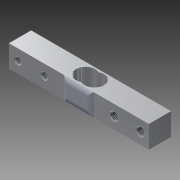
# Autodesk Inventor part: Weight Sensor
Saved by Autodesk Inventor 2014 SP1 (Build 180222100, 222)
## iProperties
Created: 2015-08-12
Part Number: Weight Sensor
Material: Алюминий 6061-AHC
Document SubType Name: Modeling
Designer: romanov.mv
Density: 2.71 g/cm^3
Appearance: Алюминий — темный
Author: romanov.mv
Autodesk Inventor part; units mm, degrees
ref_plane "YZ Plane" through (0, 0, 0) normal (1, 0, 0) x (0, 1, 0)
ref_plane "XZ Plane" through (0, 0, 0) normal (0, 1, 0) x (-1, 0, 0)
ref_plane "XY Plane" through (0, 0, 0) normal (0, 0, 1) x (1, 0, 0)
sketch "Эскиз1" plane through (0, 0, 0) normal (0, 1, 0) x (-1, 0, 0)
  line L0 (-40, 6.35) -> (40, 6.35)
  line L1 (40, 6.35) -> (40, -6.35)
  line L2 (40, -6.35) -> (-40, -6.35)
  line L3 (-40, -6.35) -> (-40, 6.35)
  line L4 (-40, 6.35) -> (40, -6.35) construction
  line L5 (40, 6.35) -> (-40, -6.35) construction
  point P0 (0, 0)
  dimension "d0" = 80
  dimension "d1" = 12.7
  constraints: 12 end point, 2 midpoint, 2 parallel, 1 horizontal, 1 perpendicular
  measures "d0" distance of L1.end L2.end
  measures "d1" distance of L0.end L1.end
extrude "Выдавливание1" add sketch "Эскиз1" along normal blind 12.7
sketch "Эскиз2" plane through (0, 12.7, 0) normal (0, 1, 0) x (1, 0, 0)
  point P0 (0, 0)
  point P1 (-35, 0)
  point P2 (-20, 0)
  point P3 (20, 0)
  point P4 (35, 0)
  dimension "d4" = 15
  dimension "d5" = 40
  dimension "d6" = 15
  dimension "d7" = 20
  measures "d4" distance of point (-20, 0) point (-35, 0)
  measures "d5" distance of point (20, 0) point (-20, 0)
  measures "d6" distance of point (35, 0) point (20, 0)
  measures "d7" distance of point (0, 0) point (-20, 0)
hole "Отверстие1" at (-35, 12.7, 0) at (-20, 12.7, 0) direction (0, -1, 0) diameter 3.242 end through all thread size "M4x0.7" class "6H" standard "ISO Metric profile"
hole "Отверстие2" at (20, 12.7, 0) at (35, 12.7, 0) direction (0, -1, 0) diameter 4.134 end through all thread size "M5x0.8" class "6H" standard "ISO Metric profile"
sketch "Эскиз3" plane through (-40, 0, 6.35) normal (0, 0, 1) x (1, 0, 0)
  line L0 (80, 0) -> (0, 0) projected
  arc A0 (40, 11.249) -> (40, 1.451) centre (37.5, 6.35) ccw
  arc A1 (40, 1.451) -> (40, 11.249) centre (42.5, 6.35) ccw
  line L1 (80, 0) -> (80, 12.7) projected
  point P0 (40, 0)
  point P1 (40, 0)
  point P2 (80, 6.35)
  dimension "d22" = 11
  dimension "d23" = 11
  dimension "d24" = 5
  constraints: 4 point on circle, 2 centre point, 2 horizontal alignment, 2 midpoint, 1 vertical alignment
  measures "d22" diameter of A0
  measures "d23" diameter of A1
  measures "d24" distance of A1.centre A0.centre
extrude "Выдавливание2" cut sketch "Эскиз3" against normal through all
sketch "Эскиз4" plane through (0, 12.7, 0) normal (0, 1, 0) x (1, 0, 0)
  line L0 (40, 6.35) -> (-40, 6.35) projected
  line L1 (-8.5, -6.35) -> (8.5, -6.35)
  line L2 (8.5, -6.35) -> (8.5, 6.35)
  line L3 (8.5, 6.35) -> (-8.5, 6.35)
  line L4 (-8.5, 6.35) -> (-8.5, -6.35)
  line L5 (-8.5, -6.35) -> (8.5, 6.35) construction
  line L6 (8.5, -6.35) -> (-8.5, 6.35) construction
  point P0 (0, 0)
  dimension "d27" = 17
  constraints: 12 end point, 2 midpoint, 2 parallel, 1 horizontal, 1 perpendicular, 1 point on line
  measures "d27" distance of L3.end L2.end
extrude "Выдавливание3" add sketch "Эскиз4" along normal blind 1 draft -50
fillet "Сопряжение1" radius 5 4 edges at (7.3082, 13.7, 0) (0, 13.7, 5.1582) (-7.3082, 13.7, 0) (0, 13.7, -5.1582)
sketch "Эскиз5" plane through (0, 0, 0) normal (0, -1, 0) x (1, 0, 0)
  line L0 (40, 6.35) -> (-40, 6.35) projected
  line L1 (-8.5, -6.35) -> (8.5, -6.35)
  line L2 (8.5, -6.35) -> (8.5, 6.35)
  line L3 (8.5, 6.35) -> (-8.5, 6.35)
  line L4 (-8.5, 6.35) -> (-8.5, -6.35)
  line L5 (-8.5, -6.35) -> (8.5, 6.35) construction
  line L6 (8.5, -6.35) -> (-8.5, 6.35) construction
  point P0 (0, 0)
  dimension "d31" = 17
  constraints: 12 end point, 2 midpoint, 2 parallel, 1 horizontal, 1 perpendicular, 1 point on line
  measures "d31" distance of L3.end L2.end
extrude "Выдавливание4" add sketch "Эскиз5" along normal blind 1 draft -50
fillet "Сопряжение2" radius 5 4 edges at (-7.3082, -1, 0) (0, -1, 5.1582) (7.3082, -1, 0) (0, -1, -5.1582)
chamfer "Фаска1" distance 0.5 angle 45 8 edges at (-35, 12.7, -1.621) (-20, 12.7, -1.621) (20, 12.7, -2.067) (35, 12.7, -2.067) (20, 0, -2.067) (35, 0, -2.067) (-20, 0, -1.621) (-35, 0, -1.621)
